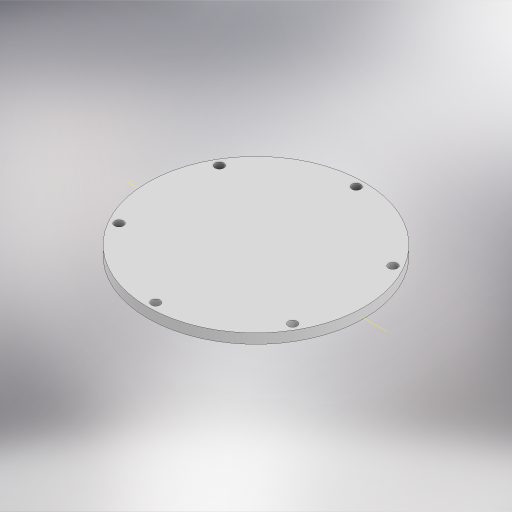
# Autodesk Inventor part: Deckel Stempel 2
Saved by Autodesk Inventor 2023 (Build 270158000, 158)
## iProperties
Created: 2022-11-23
Part Number: Deckel Stempel 2
Material: Generisch
Document SubType Name: Modeling
Designer: schil
Density: 1 g/cm^3
Appearance: Vorgabe
Author: schil
Autodesk Inventor part; units mm, degrees
ref_plane "YZ Plane" through (0, 0, 0) normal (1, 0, 0) x (0, 1, 0)
ref_plane "XZ Plane" through (0, 0, 0) normal (0, 1, 0) x (-1, 0, 0)
ref_plane "XY Plane" through (0, 0, 0) normal (0, 0, 1) x (1, 0, 0)
sketch "Skizze1" plane through (0, 0, 0) normal (1, 0, 0) x (0, 1, 0)
  line L0 (5, -20) -> (5, -25)
  line L1 (5, -20) -> (0, -20)
  line L2 (0, -20) -> (0, -55)
  line L3 (0, -55) -> (5, -55)
  line L4 (5, -55) -> (5, -20)
  line L5 (0, -42) -> (0, -47)
  line L6 (0, -37.5) -> (0, -42)
  line L7 (-8, 0) -> (13, 0) projected
  line L8 (0, -66) -> (0, 11) projected
  line L9 (5, -20) -> (0, -20)
  line L10 (0, -20) -> (0, 0)
  line L11 (0, 0) -> (5, 0)
  line L12 (5, 0) -> (5, -20)
  line L13 (-5, 0) -> (0, 0)
  line L14 (0, 0) -> (0, -47)
  line L15 (0, -47) -> (-5, -47)
  line L16 (-5, -47) -> (-5, 0)
  point P0 (10, -25)
  point P1 (10, -20)
  point P2 (0, -44.5)
  point P3 (2.5, -55)
  point P4 (-2.5, -47)
  dimension "d1" = 5
  dimension "d10" = 0
  dimension "d26" = 5
  dimension "d27" = 47
  constraints: 30 end point, 6 parallel, 3 horizontal, 3 midpoint, 3 perpendicular, 3 point on line
  measures "d1" distance from line of point (0, -44.5) L4
  measures "d10" distance between parallel lines of L8 L2
  measures "d26" distance between parallel lines of L14 L16
  measures "d27" distance from line of L7 point (-2.5, -47)
revolve "Umdrehung1" add sketch "Skizze1" angle 360 about axis through (0, -10, 0) along (0, 1, 0)
sketch "Skizze2" plane through (0, 5, 0) normal (0, 1, 0) x (1, 0, 0)
  line L0 (-77, 0) -> (77, 0) projected
  line L1 (0, 77) -> (0, -77) projected
  circle A0 centre (0, 0) radius 51
  circle A1 centre (0, 0) radius 55 projected
  point P0 (0, -51)
  point P1 (44.1673, -25.5)
  point P2 (44.1673, 25.5)
  point P3 (0, 51)
  point P4 (-44.1673, 25.5)
  point P5 (-44.1673, -25.5)
  dimension "d14" = 4
  dimension "d17" = 360
  constraints: 1 coincident, 1 point on line, 1 vertical alignment, 9 other
hole "Bohrung1" at (0, 5, 51) at (44.1673, 5, 25.5) at (44.1673, 5, -25.5) at (0, 5, -51) at (-44.1673, 5, -25.5) at (-44.1673, 5, 25.5) direction (0, -1, 0) diameter 4.5 depth 11.8 tip angle 118
